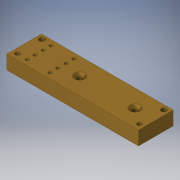
# Autodesk Inventor part: OneTalonSRXPlateTwo
Saved by Autodesk Inventor 2019 (Build 230136000, 136)
## iProperties
Created: 2017-09-23
Part Number: OneTalonSRXPlateTwo
Material: Generic
Document SubType Name: Modeling
Designer: james
Density: 1 g/cm^3
Appearance: Brass - Satin
Author: james
Autodesk Inventor part; units mm, degrees
ref_plane "YZ Plane" through (0, 0, 0) normal (1, 0, 0) x (0, 1, 0)
ref_plane "XZ Plane" through (0, 0, 0) normal (0, 1, 0) x (-1, 0, 0)
ref_plane "XY Plane" through (0, 0, 0) normal (0, 0, 1) x (1, 0, 0)
sketch "Sketch1" plane through (0, 0, 0) normal (0, 1, 0) x (-1, 0, 0)
  line L0 (46.6228, 34.6302) -> (-74.0272, 34.6302)
  line L1 (-74.0272, 34.6302) -> (-74.0272, -28.8698)
  line L2 (-74.0272, -28.8698) -> (46.6228, -28.8698)
  line L3 (46.6228, -28.8698) -> (46.6228, 34.6302)
  point P0 (0, 0)
  dimension "d0" = 120.65
  dimension "d1" = 63.5
  constraints: 8 end point, 2 parallel, 1 horizontal, 1 perpendicular
  measures "d0" distance of L0.start L0.end
  measures "d1" distance of L2.end L0.start
extrude "Extrusion1" add sketch "Sketch1" along normal blind 12.7
sketch "Sketch4" plane through (0, 0, 0) normal (0, -1, 0) x (1, 0, 0)
  line L0 (74.0272, -28.8698) -> (-46.6228, -28.8698) projected
  line L1 (-28.8428, 23.5502) -> (-28.8428, 29.5502) projected
  line L2 (-46.6228, -28.8698) -> (-46.6228, 34.6302) projected
  point P0 (0, 0)
  point P1 (-32.8428, -16.6898)
  point P2 (-32.8428, -23.7898)
  point P3 (-11.9428, -23.7898)
  point P4 (-11.9428, -16.6898)
  dimension "d21" = 0
  dimension "d22" = 0
  dimension "d23" = 0
  dimension "d24" = 0
  dimension "d25" = 5.08
  dimension "d26" = 7.1
  dimension "d27" = 20.9
  dimension "d35" = 4
  dimension "d92" = 13.78
  measures "d21" horizontal distance of point (-11.943, -16.69) point (-11.943, -23.79)
  measures "d22" vertical distance of point (-32.843, -16.69) point (-11.943, -16.69)
  measures "d23" vertical distance of point (-32.843, -23.79) point (-11.943, -23.79)
  measures "d24" horizontal distance of point (-32.843, -16.69) point (-32.843, -23.79)
  measures "d25" distance from line of L0 point (-11.943, -23.79)
  measures "d26" distance of point (-32.843, -16.69) point (-32.843, -23.79)
  measures "d27" distance of point (-11.943, -16.69) point (-32.843, -16.69)
  measures "d35" distance from line of point (-32.843, -23.79) L1
  measures "d92" distance from line of point (-32.843, -23.79) L2
hole "Hole2" at (-32.8428, 0, -16.6898) at (-32.8428, 0, -23.7898) at (-11.9428, 0, -23.7898) at (-11.9428, 0, -16.6898) direction (0, 1, 0) diameter 2.8 depth 25.4 tip angle 118
sketch "Sketch6" plane through (0, 0, 0) normal (0, -1, 0) x (1, 0, 0)
  line L0 (-46.6228, 34.6302) -> (74.0272, 34.6302) projected
  line L1 (-46.6228, -28.8698) -> (-46.6228, 34.6302) projected
  line L2 (74.0272, -28.8698) -> (-46.6228, -28.8698) projected
  point P0 (0, 0)
  point P1 (69.7092, -24.6788)
  point P2 (-42.0508, -24.6788)
  point P3 (-42.0508, 30.4392)
  point P4 (69.7092, 30.4392)
  dimension "d43" = 0
  dimension "d44" = 0
  dimension "d46" = 111.76
  dimension "d47" = 0
  dimension "d48" = 0
  dimension "d50" = 4.191
  dimension "d51" = 4.572
  dimension "d91" = 4.191
  measures "d43" horizontal distance of point (69.709, -24.679) point (69.709, 30.439)
  measures "d44" vertical distance of point (-42.051, 30.439) point (69.709, 30.439)
  measures "d46" distance of point (69.709, 30.439) point (-42.051, 30.439)
  measures "d47" horizontal distance of point (-42.051, 30.439) point (-42.051, -24.679)
  measures "d48" vertical distance of point (69.709, -24.679) point (-42.051, -24.679)
  measures "d50" distance from line of L0 point (-42.051, 30.439)
  measures "d51" distance from line of L1 point (-42.051, 30.439)
  measures "d91" distance from line of L2 point (-42.051, -24.679)
hole "Hole4" at (69.7092, 0, -24.6788) at (-42.0508, 0, -24.6788) at (-42.0508, 0, 30.4392) at (69.7092, 0, 30.4392) direction (0, 1, 0) diameter 4.8 depth 25.4 tip angle 118
sketch "Sketch10" plane through (0, 12.7, 0) normal (0, 1, 0) x (1, 0, 0)
  circle A0 centre (54.9772, -18.7552) radius 2.413 projected
  circle A1 centre (4.1772, -18.7552) radius 2.413 projected
  line L0 (74.0272, 28.8698) -> (-46.6228, 28.8698) projected
  point P0 (0, 0)
  point P1 (4.1772, 12.9948)
  point P2 (54.9772, 12.9948)
  point P3 (66.6772, 28.8698)
  point P4 (-45.6228, 28.8698)
  dimension "d80" = 0
  dimension "d81" = 0
  dimension "d82" = 0
  dimension "d83" = 15.875
  measures "d80" horizontal distance of A1.centre point (4.177, 12.995)
  measures "d81" horizontal distance of point (54.977, 12.995) A0.centre
  measures "d82" vertical distance of point (4.177, 12.995) point (54.977, 12.995)
  measures "d83" distance from line of L0 point (4.177, 12.995)
hole "Hole7" at (4.1772, 12.7, -12.9948) at (54.9772, 12.7, -12.9948) direction (0, -1, 0) diameter 4.826 end through all countersink diameter 9.525 countersink angle 82
sketch "Sketch11" plane through (0, 0, 0) normal (0, -1, 0) x (1, 0, 0)
  line L0 (-28.8428, -3.0578) -> (-16.8428, -3.0578)
  line L1 (-16.8428, -3.0578) -> (-16.8428, -9.0578)
  line L2 (-16.8428, -9.0578) -> (-28.8428, -9.0578)
  line L3 (-28.8428, -9.0578) -> (-28.8428, -3.0578)
  line L4 (-28.8428, -17.7898) -> (-16.8428, -17.7898)
  line L5 (-16.8428, -17.7898) -> (-16.8428, -23.7898)
  line L6 (-16.8428, -23.7898) -> (-28.8428, -23.7898)
  line L7 (-28.8428, -23.7898) -> (-28.8428, -17.7898)
  line L8 (-28.8428, 23.5502) -> (-28.8428, 29.5502) projected
  line L9 (-16.8428, 29.5502) -> (-16.8428, 23.5502) projected
  line L10 (74.0272, -28.8698) -> (-46.6228, -28.8698) projected
  point P0 (0, 0)
  dimension "d93" = 0
  dimension "d94" = 0
  dimension "d95" = 0
  dimension "d96" = 0
  dimension "d97" = 6
  dimension "d98" = 6
  dimension "d99" = 5.08
  dimension "d100" = 19.812
  constraints: 16 end point, 4 parallel, 2 horizontal, 2 perpendicular
  measures "d93" distance between parallel lines of L3 L8
  measures "d94" distance between parallel lines of L9 L1
  measures "d95" distance between parallel lines of L1 L5
  measures "d96" distance between parallel lines of L3 L7
  measures "d97" distance of L2.end L0.start
  measures "d98" distance of L6.end L4.start
  measures "d99" distance between parallel lines of L10 L6
  measures "d100" distance between parallel lines of L2 L10
extrude "Extrusion4" cut sketch "Sketch11" against normal blind 1.27
sketch "Sketch12" plane through (0, 0, 0) normal (0, -1, 0) x (1, 0, 0)
  circle A0 centre (-42.0508, 30.4392) radius 2.4 projected
  circle A1 centre (69.7092, 30.4392) radius 2.4 projected
  circle A2 centre (69.7092, -24.6788) radius 2.4 projected
  circle A3 centre (-42.0508, -24.6788) radius 2.4 projected
  point P0 (0, 0)
  constraints: 4 coincident
hole "Hole8" at (-42.0508, 0, 30.4392) at (69.7092, 0, 30.4392) at (69.7092, 0, -24.6788) at (-42.0508, 0, -24.6788) direction (0, 1, 0) diameter 4.826 end through all
sketch "Sketch13" plane through (0, 0, 0) normal (0, -1, 0) x (1, 0, 0)
  circle A0 centre (-32.8428, -16.6898) radius 1.4 projected
  circle A1 centre (-32.8428, -23.7898) radius 1.4 projected
  circle A2 centre (-11.9428, -16.6898) radius 1.4 projected
  point P0 (0, 0)
  point P1 (-32.8428, -9.0698)
  point P2 (-32.8428, -1.9578)
  point P3 (-39.7887, 34.6302)
  point P4 (67.4471, 34.6302)
  point P5 (-11.9428, -9.0698)
  point P6 (-11.9428, -1.9578)
  dimension "d112" = 0
  dimension "d113" = 7.112
  dimension "d115" = 7.62
  dimension "d117" = 0
  dimension "d120" = 0
  dimension "d123" = 0
  dimension "d124" = 0
  measures "d112" horizontal distance of point (-32.843, -1.958) point (-32.843, -9.07)
  measures "d113" distance of point (-32.843, -1.958) point (-32.843, -9.07)
  measures "d115" distance of point (-32.843, -9.07) A0.centre
  measures "d117" horizontal distance of point (-11.943, -1.958) point (-11.943, -9.07)
  measures "d120" horizontal distance of A2.centre point (-11.943, -9.07)
  measures "d123" vertical distance of point (-32.843, -1.958) point (-11.943, -1.958)
  measures "d124" vertical distance of point (-32.843, -9.07) point (-11.943, -9.07)
hole "Hole9" at (-32.8428, 0, -9.0698) at (-32.8428, 0, -1.9578) at (-11.9428, 0, -9.0698) at (-11.9428, 0, -1.9578) direction (0, 1, 0) diameter 2.8 end through all
sketch "Sketch15" plane through (0, 12.7, 0) normal (0, 1, 0) x (1, 0, 0)
  circle A0 centre (4.1772, -18.7552) radius 2.413 projected
  circle A1 centre (54.9772, -18.7552) radius 2.413 projected
  circle A2 centre (4.1772, -18.7552) radius 3.3734
  circle A3 centre (54.9772, -18.7552) radius 3.3734
  point P0 (0, 0)
  point P1 (4.1772, 12.9948)
  point P2 (54.9772, 12.9948)
  dimension "d140" = 6.7469
  dimension "d141" = 6.7469
  constraints: 2 centre point, 2 coincident
  measures "d140" diameter of A3
  measures "d141" diameter of A2
extrude "Extrusion6" [suppressed]
sketch "Sketch16" plane through (0, 0, 0) normal (0, -1, 0) x (1, 0, 0)
  line L0 (-74.1492, 48.5934) -> (104.9801, 48.5934)
  line L1 (104.9801, 48.5934) -> (104.9801, 2.8802)
  line L2 (104.9801, 2.8802) -> (-74.1492, 2.8802)
  line L3 (-74.1492, 2.8802) -> (-74.1492, 48.5934)
  line L4 (-46.6228, 34.6302) -> (74.0272, 34.6302) projected
  point P0 (0, 0)
  dimension "d157" = 31.75
  constraints: 8 end point, 2 parallel, 1 horizontal, 1 perpendicular
  measures "d157" distance between parallel lines of L2 L4
extrude "Extrusion7" cut sketch "Sketch16" against normal blind 25.4
sketch "Sketch17" plane through (0, 0, 0) normal (0, -1, 0) x (1, 0, 0)
  line L0 (74.0272, 2.8802) -> (-46.6228, 2.8802) projected
  line L1 (-46.6228, -28.8698) -> (-46.6228, 2.8802) projected
  line L2 (74.0272, -28.8698) -> (-46.6228, -28.8698) projected
  line L3 (74.0272, 2.8802) -> (74.0272, -28.8698) projected
  circle A0 centre (-11.9428, -9.0698) radius 1.4 projected
  circle A1 centre (-32.8428, -9.0698) radius 1.4 projected
  circle A2 centre (-32.8428, -1.9578) radius 1.4 projected
  circle A3 centre (-11.9428, -1.9578) radius 1.4 projected
  circle A4 centre (69.7092, -24.6788) radius 2.413 projected
  circle A5 centre (-42.0508, -24.6788) radius 2.413 projected
  line L4 (-28.8428, -9.0578) -> (-28.8428, -3.0578) projected
  line L5 (-28.8428, -3.0578) -> (-16.8428, -3.0578) projected
  line L6 (-16.8428, -3.0578) -> (-16.8428, -9.0578) projected
  line L7 (-16.8428, -9.0578) -> (-28.8428, -9.0578) projected
  line L8 (-28.8428, -23.7898) -> (-28.8428, -17.7898) projected
  line L9 (-28.8428, -17.7898) -> (-16.8428, -17.7898) projected
  line L10 (-16.8428, -17.7898) -> (-16.8428, -23.7898) projected
  line L11 (-16.8428, -23.7898) -> (-28.8428, -23.7898) projected
  circle A6 centre (4.1772, -12.9948) radius 2.413 projected
  circle A7 centre (54.9772, -12.9948) radius 2.413 projected
  circle A8 centre (-11.9428, -23.7898) radius 1.4 projected
  circle A9 centre (-32.8428, -16.6898) radius 1.4 projected
  circle A10 centre (-32.8428, -23.7898) radius 1.4 projected
  circle A11 centre (-11.9428, -16.6898) radius 1.4 projected
  circle A12 centre (-42.0508, -24.6788) radius 2.413 projected
  point P0 (0, 0)
  point P1 (-42.0508, -2.1998)
  point P2 (69.7092, -2.1998)
  dimension "d146" = 0
  dimension "d147" = 0
  dimension "d148" = 0
  dimension "d149" = 5.08
  measures "d146" vertical distance of point (69.709, -2.2) point (-42.051, -2.2)
  measures "d147" horizontal distance of A5.centre point (-42.051, -2.2)
  measures "d148" horizontal distance of A4.centre point (69.709, -2.2)
  measures "d149" distance from line of L0 point (-42.051, -2.2)
hole "Hole10" at (-42.0508, 0, -2.1998) at (69.7092, 0, -2.1998) direction (0, 1, 0) diameter 3.9624 end through all thread size "10-32 UNF" class "2B" standard "ANSI Unified Screw Threads"
equation "\"d1\" = 2 * TalonSRXWidth"
equation "\"d26\" = CanConBetweenTopHoles"
equation "\"d27\" = CanConBetweenSideHoles"
equation "\"d35\" = CanConHoleFromTopPin"
equation "\"d28\" = CanConHoleDiam"
equation "\"d52\" = LegoMainHole"
equation "\"d83\" = TalonSRXFromSide"
equation "\"d125\" = CanConHoleDiam"
equation "\"LegoMainHole\" = 4.8"
equation "\"TalonSRXWidth\" = 31.75"
equation "\"TalonSRXFromSide\" = 15.875"
equation "\"TalonSRXBetweenHoles\" = 50.8"
equation "\"CanConPinWidth\" = 6"
equation "\"CanConPinLength\" = 12"
equation "\"CanConBetweenSideHoles\" = 20.9"
equation "\"CanConBetweenTopHoles\" = 7.1"
equation "\"CanConHoleDiam\" = 2.8"
equation "\"CanConHoleFromTopPin\" = 4"
body "Solid1"
